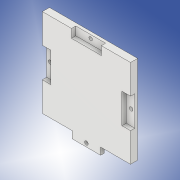
# Autodesk Inventor part: TC007
Saved by Autodesk Inventor 2017 SP1 (Build 210196100, 196)
## iProperties
Created: 2017-08-15
Part Number: TC007
Material: ABS Plastic
Document SubType Name: Modeling
Designer: Zach
Density: 1.06 g/cm^3
Appearance: CR White
Author: Zach
Autodesk Inventor part; units mm, degrees
ref_plane "YZ Plane" through (0, 0, 0) normal (1, 0, 0) x (0, 1, 0)
ref_plane "XZ Plane" through (0, 0, 0) normal (0, 1, 0) x (-1, 0, 0)
ref_plane "XY Plane" through (0, 0, 0) normal (0, 0, 1) x (1, 0, 0)
sketch "Sketch1" plane through (0, 0, 0) normal (0, 0, 1) x (1, 0, 0)
  line L0 (0, 0) -> (124, 0)
  line L1 (124, 0) -> (124, 124)
  line L2 (124, 124) -> (0, 124)
  line L3 (0, 124) -> (0, 0)
  circle A0 centre (5, 62) radius 2.5
  circle A1 centre (119, 62) radius 2.5
  circle A2 centre (62, 119) radius 2.5
  point P0 (124, 62)
  point P1 (0, 62)
  point P2 (62, 124)
  dimension "d0" = 124
  dimension "d1" = 124
  dimension "d2" = 5
  dimension "d3" = 5
  dimension "d4" = 5
  dimension "d5" = 5
  dimension "d6" = 5
  dimension "d7" = 5
  constraints: 8 end point, 3 centre point, 3 horizontal alignment, 3 midpoint, 2 parallel, 1 horizontal, 1 perpendicular, 1 vertical alignment
  measures "d0" distance of L2.end L1.end
  measures "d1" distance of L1.end L0.end
  measures "d2" diameter of A0
  measures "d3" diameter of A1
  measures "d4" distance of point (0, 62) A0.centre
  measures "d5" distance of point (124, 62) A1.centre
  measures "d6" diameter of A2
  measures "d7" distance of point (62, 124) A2.centre
extrude "Extrusion1" add sketch "Sketch1" along normal blind 10
sketch "Sketch2" plane through (0, 0, 10) normal (0, 0, 1) x (1, 0, 0)
  line L0 (0, 83) -> (12, 83)
  line L1 (12, 83) -> (12, 41)
  line L2 (12, 41) -> (0, 41)
  line L3 (0, 41) -> (0, 83)
  line L4 (124, 124) -> (0, 124) projected
  line L5 (41, 124) -> (83, 124)
  line L6 (83, 124) -> (83, 112)
  line L7 (83, 112) -> (41, 112)
  line L8 (41, 112) -> (41, 124)
  line L9 (124, 0) -> (124, 124) projected
  line L10 (124, 83) -> (112, 83)
  line L11 (112, 83) -> (112, 41)
  line L12 (112, 41) -> (124, 41)
  line L13 (124, 41) -> (124, 83)
  line L14 (0, 124) -> (0, 0) projected
  point P0 (62, 112)
  point P1 (62, 124)
  point P2 (112, 62)
  point P3 (124, 62)
  point P4 (12, 62)
  point P5 (0, 62)
  dimension "d10" = 12
  dimension "d11" = 42
  dimension "d12" = 42
  dimension "d13" = 12
  dimension "d14" = 12
  dimension "d15" = 42
  constraints: 24 end point, 6 midpoint, 6 parallel, 3 horizontal, 3 perpendicular, 2 horizontal alignment, 2 point on line, 2 vertical alignment
  measures "d10" distance of L1.end L2.end
  measures "d11" distance of L0.end L1.end
  measures "d12" distance of L6.end L7.end
  measures "d13" distance of L5.end L6.end
  measures "d14" distance of L12.end L11.end
  measures "d15" distance of L11.end L10.end
extrude "Extrusion2" cut sketch "Sketch2" against normal blind 6
sketch "Sketch3" plane through (0, 0, 10) normal (0, 0, 1) x (1, 0, 0)
  line L0 (0, 0) -> (124, 0) projected
  line L1 (42, 0) -> (82, 0)
  line L2 (82, 0) -> (82, -10)
  line L3 (82, -10) -> (42, -10)
  line L4 (42, -10) -> (42, 0)
  circle A0 centre (62, -5) radius 2.5
  point P0 (42, -5)
  point P1 (62, -10)
  point P2 (62, 0)
  point P3 (62, 0)
  dimension "d18" = 40
  dimension "d19" = 10
  dimension "d20" = 5
  constraints: 8 end point, 4 midpoint, 2 parallel, 1 centre point, 1 coincident, 1 horizontal, 1 horizontal alignment, 1 perpendicular, 1 point on line, 1 vertical alignment
  measures "d18" distance of L2.end L3.end
  measures "d19" distance of L1.end L2.end
  measures "d20" diameter of A0
extrude "Extrusion3" add sketch "Sketch3" against normal blind 5
body "Solid1"
